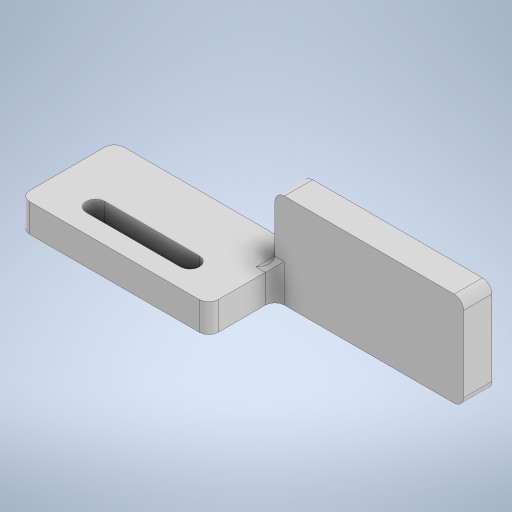
# Autodesk Inventor part: servo attachment
Saved by Autodesk Inventor 2023 (Build 270158000, 158)
## iProperties
Created: 2023-03-30
Part Number: servo attachment
Material: Generic
Document SubType Name: Modeling
Designer: Steven
Density: 1 g/cm^3
Appearance: Default
Author: Steven
Autodesk Inventor part; units mm, degrees
ref_plane "YZ Plane" through (0, 0, 0) normal (1, 0, 0) x (0, 1, 0)
ref_plane "XZ Plane" through (0, 0, 0) normal (0, 1, 0) x (-1, 0, 0)
ref_plane "XY Plane" through (0, 0, 0) normal (0, 0, 1) x (1, 0, 0)
sketch "Sketch1" plane through (0, 0, 0) normal (0, 1, 0) x (-1, 0, 0)
  line L0 (0, 0) -> (-20, 0)
  line L1 (-20, 0) -> (-20, -10)
  line L2 (-20, -10) -> (0, -10)
  line L3 (0, -10) -> (0, 0)
  line L4 (-15, -3) -> (-5, -3) construction
  line L5 (-15, -4) -> (-5, -4)
  line L6 (-5, -2) -> (-15, -2)
  arc A0 (-15, -2) -> (-15, -4) centre (-15, -3) ccw
  arc A1 (-5, -4) -> (-5, -2) centre (-5, -3) ccw
  point P0 (-10, -3)
  point P1 (-10, -10)
  point P2 (-20, -5)
  dimension "d0" = 20
  dimension "d1" = 10
  dimension "d2" = 2
  dimension "d3" = 10
  dimension "d10" = 2
  constraints: 16 end point, 4 point on circle, 4 tangent, 3 midpoint, 3 parallel, 2 centre point, 2 horizontal, 1 perpendicular, 1 vertical alignment
  measures "d0" distance of L2.end L1.end
  measures "d1" distance of L0.end L1.end
  measures "d2" diameter of A1
  measures "d3" distance of L5.start L5.end
  measures "d10" distance between parallel lines of L0 L6
extrude "Extrusion1" add sketch "Sketch1" along normal blind 3
sketch "Sketch2" plane through (20, 0, -10) normal (0, 0, -1) x (-1, 0, 0)
  line L0 (0, 0) -> (0, 3) projected
  line L1 (0, 0) -> (-20, 0)
  line L2 (-20, 0) -> (-20, 10)
  line L3 (-20, 10) -> (0, 10)
  line L4 (0, 10) -> (0, 0)
  point P0 (20, 0)
  point P1 (0, 3)
  dimension "d6" = 10
  dimension "d7" = 20
  constraints: 8 end point, 2 parallel, 1 horizontal, 1 perpendicular
  measures "d6" distance of L1.end L2.end
  measures "d7" distance of L2.end L3.end
extrude "Extrusion2" add sketch "Sketch2" against normal blind 3
fillet "Fillet1" radius 1 5 edges at (0, 1.5, -10) (0, 1.5, 0) (20, 1.5, 0) (20, 3, -8.5) (20, 1.5, -7)
fillet "Fillet2" radius 1 2 edges at (19.5, 3, -7) (20.5, 3, -7)
fillet "Fillet3" radius 1 3 edges at (20, 10, -8.5) (40, 10, -8.5) (40, 0, -8.5)
body "Solid1"
